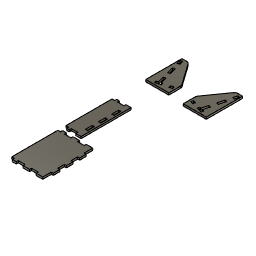
socle_carte_makers_quest_v5 (Autodesk Fusion 360 design; units mm, degrees)
Autodesk Fusion 360 part; units mm, degrees
sketch "Esquisse1" plane through (0, 0, 0) normal (0, 1, 0) x (1, 0, 0)
  line L0 (0, 0) -> (35, 0)
  line L1 (35, 0) -> (35, -55)
  line L2 (35, -55) -> (0, -55)
  line L3 (0, -55) -> (0, 0)
  line L4 (0, -55) -> (12.941, -6.7037)
  line L5 (0, -55) -> (50, -55) construction
  line L6 (12.941, -6.7037) -> (35, -12.6144)
  line L7 (12.941, -6.7037) -> (15.8387, -7.4802)
  line L8 (15.8387, -7.4802) -> (2.8978, -55.7765)
  line L9 (2.8978, -55.7765) -> (0, -55)
  line L10 (0, -55) -> (12.941, -6.7037)
  line L11 (35, -12.6144) -> (35.7765, -9.7166)
  line L12 (35.7765, -9.7166) -> (13.7176, -3.806)
  line L13 (13.7176, -3.806) -> (12.9412, -6.7038)
  line L14 (12.9412, -6.7038) -> (35, -12.6144)
  dimension "d1" = 35
  dimension "d2" = 55
  dimension "d3" = 75
  dimension "d4" = 50
  dimension "d5" = 3
  dimension "d6" = 50
  dimension "d7" = 22.8372
  dimension "d8" = 3
  dimension "d9" = 22.837
  constraint horizontal L0
  constraint vertical L1
  constraint horizontal L2
  constraint vertical L3
  constraint coincident L0.start L3.end
  constraint horizontal L5
  constraint coincident L1 L6.end
  constraint perpendicular L4 L6
  constraint parallel L4 L10
  constraint parallel L6 L14
  measures "d1" distance of L0.start L0.end
  measures "d2" distance of L0.start L2.end
  measures "d3" angle of L4 L5
  measures "d4" distance of L2.end L4.end
  measures "d5" distance of L4.end L7.end
  measures "d6" distance of L4.end L2.end
  measures "d7" distance of L4.end L6.end
  measures "d8" distance of L6.end L11.end
  measures "d9" distance of L6.end L13.end
extrude "Extrusion1" add sketch "Esquisse1" along normal blind 70 contours L1 L11 L12 | L1 L6 L7 L12 L13 L14 makes body 1
extrude "Extrusion2" add sketch "Esquisse1" along normal blind 70 separate body contours L2 L4 L6 L7 L8 L10 L14 | L2 L8 L9 makes body 2
extrude "Extrusion3" add sketch "Esquisse1" against normal blind 3 separate body contours L0 L1 L3 L4 L10 L12 L13 | L2 L4 L6 L7 L8 L10 L14 | L1 L6 L7 L12 L13 L14 | L1 L2 L6 L8 L14 makes body 3
copy_body "Copier/Coller des corps1" bodies 3 makes body 4
move_body "Déplacer1" bodies 4 to x (1, 0, 0) y (0, 1, 0) z (0, 0, 1) at (0, 73, 0)
extrude "Extrusion5" add 1 faces at (13.4587, 23.3333, 4.7719) along direction (-0.965926, 0, -0.258819) blind 3 on bodies 1 bodies 1
sketch "Esquisse2" plane through (-0.809, 0, 3.0194) normal (0.258819, 0, -0.965926) x (0, 1, 0)
  line L0 (0, 17.235) -> (0, 14.235)
  line L1 (0, 14.235) -> (70, 14.235)
  line L2 (70, 14.235) -> (70, 17.235)
  line L3 (70, 17.235) -> (0, 17.235)
  line L4 (0, 17.235) -> (10, 17.235) construction
  line L5 (10, 17.235) -> (10, 14.235) construction
  line L6 (10, 14.235) -> (0, 14.235) construction
  line L7 (0, 14.235) -> (0, 17.235) construction
  line L8 (70, 17.235) -> (60, 17.235) construction
  line L9 (60, 17.235) -> (60, 14.235) construction
  line L10 (60, 14.235) -> (70, 14.235) construction
  line L11 (70, 14.235) -> (70, 17.235) construction
  line L12 (10, 17.235) -> (20, 17.235)
  line L13 (20, 17.235) -> (20, 14.235)
  line L14 (20, 14.235) -> (10, 14.235)
  line L15 (10, 14.235) -> (10, 17.235)
  line L16 (60, 17.235) -> (50, 17.235)
  line L17 (50, 17.235) -> (50, 14.235)
  line L18 (50, 14.235) -> (60, 14.235)
  line L19 (60, 14.235) -> (60, 17.235)
  line L20 (20, 17.235) -> (30, 17.235) construction
  line L21 (30, 17.235) -> (30, 14.235) construction
  line L22 (30, 14.235) -> (20, 14.235) construction
  line L23 (20, 14.235) -> (20, 17.235) construction
  line L24 (30, 17.235) -> (40, 17.235)
  line L25 (40, 17.235) -> (40, 14.235)
  line L26 (40, 14.235) -> (30, 14.235)
  line L27 (30, 14.235) -> (30, 17.235)
  dimension "d20" = 10
  dimension "d21" = 10
  dimension "d22" = 10
  dimension "d23" = 10
  dimension "d24" = 10
  dimension "d25" = 10
  constraint horizontal L4
  constraint vertical L5
  constraint horizontal L6
  constraint vertical L7
  constraint coincident L0.start L3.end
  constraint horizontal L8
  constraint vertical L9
  constraint horizontal L10
  constraint vertical L11
  constraint coincident L2.end L3.start
  constraint horizontal L12
  constraint vertical L13
  constraint horizontal L14
  constraint vertical L15
  constraint horizontal L16
  constraint vertical L17
  constraint horizontal L18
  constraint vertical L19
  constraint horizontal L20
  constraint vertical L21
  constraint horizontal L22
  constraint vertical L23
  constraint horizontal L24
  constraint vertical L25
  constraint horizontal L26
  constraint vertical L27
  measures "d20" distance of L0.start L4.end
  measures "d21" distance of L2.end L8.end
  measures "d22" distance of L4.end L12.end
  measures "d23" distance of L8.end L16.end
  measures "d24" distance of L12.end L20.end
  measures "d25" distance of L20.end L24.end
extrude "Extrusion6" add sketch "Esquisse2" along normal blind 3 contours L1 L3 L12 L13 L14 L15 | L1 L3 L24 L25 L26 L27 | L1 L3 L16 L17 L18 L19 bodies 2
combine "Combiner1" operation cut target body 1 tool bodies 2 keep tools
sketch "Esquisse3" plane through (0, 70, 0) normal (0, 1, 0) x (-1, 0, 0)
  line L0 (-10.0434, 5.9273) -> (-35, 12.6144)
  line L1 (-35, 12.6144) -> (-35.7765, 9.7166)
  line L2 (-35.7765, 9.7166) -> (-10.8198, 3.0295)
  line L3 (-10.8198, 3.0295) -> (-10.0434, 5.9273)
  line L4 (-12.941, 6.7037) -> (0, 55)
  line L5 (0, 55) -> (-2.8978, 55.7765)
  line L6 (-2.8978, 55.7765) -> (-15.8387, 7.4802)
  line L7 (-15.8387, 7.4802) -> (-12.941, 6.7037)
  line L8 (-35, 12.6144) -> (-27.2726, 10.5439)
  line L9 (-27.2726, 10.5439) -> (-28.0491, 7.6461)
  line L10 (-28.0491, 7.6461) -> (-35.7765, 9.7166)
  line L11 (-35.7765, 9.7166) -> (-35, 12.6144)
  line L12 (-10.8198, 3.0295) -> (-18.5472, 5.1001)
  line L13 (0, 55) -> (-2.8978, 55.7765)
  line L14 (-2.5882, 45.3407) -> (0, 55)
  line L15 (-15.8387, 7.4802) -> (-12.941, 6.7037)
  line L16 (-12.941, 6.7037) -> (-10.3528, 16.363)
  line L17 (-10.3528, 16.363) -> (-13.2505, 17.1394)
  line L18 (-13.2505, 17.1394) -> (-15.8387, 7.4802)
  line L19 (-13.2505, 17.1394) -> (-10.3528, 16.363) construction
  line L20 (-2.8978, 55.7765) -> (-5.486, 46.1172)
  line L21 (-5.486, 46.1172) -> (-2.5882, 45.3407)
  line L22 (-8.0742, 36.4579) -> (-10.6623, 26.7987)
  line L23 (-10.6623, 26.7987) -> (-7.7646, 26.0222)
  line L24 (-8.0742, 36.4579) -> (-5.1764, 35.6815)
  line L25 (-5.1764, 35.6815) -> (-7.7646, 26.0222)
  line L26 (-10.8198, 3.0295) -> (-10.0434, 5.9273)
  line L27 (-10.0434, 5.9273) -> (-17.7708, 7.9979)
  line L28 (-17.7708, 7.9979) -> (-18.5472, 5.1001)
  line L29 (-3.9331, 51.9128) -> (-1.0353, 51.1363)
  line L30 (-31.1363, 11.5791) -> (-31.9128, 8.6814)
  point P0 (-8.0742, 36.4579)
  dimension "d28" = 8
  dimension "d29" = 3
  dimension "d30" = 8
  dimension "d32" = 3
  dimension "d33" = 10
  dimension "d34" = 3
  dimension "d35" = 10
  dimension "d38" = 3
  dimension "d42" = 10
  dimension "d43" = 10
  dimension "d44" = 10
  dimension "d45" = 8
  dimension "d50" = 3
  dimension "d51" = 4
  dimension "d52" = 4
  constraint coincident L0.end L1.start
  constraint parallel L2 L10
  constraint coincident L2.end L3.start
  constraint parallel L0 L12
  constraint coincident L4.end L5.start
  constraint coincident L6.end L7.start
  constraint parallel L4 L16
  constraint parallel L4 L14
  constraint perpendicular L13 L20
  constraint coincident L6 P0
  constraint coincident P0 L22.start
  constraint parallel L6 L22
  constraint coincident L4 L23.end
  constraint perpendicular L4 L23
  constraint coincident L4 L24.end
  constraint perpendicular L4 L24
  constraint coincident L0.start L3.end
  constraint perpendicular L26 L27
  constraint coincident L20 L29.start
  constraint coincident L6 L29.start
  constraint perpendicular L14 L29
  constraint perpendicular L20 L29
  constraint coincident L8 L30.start
  constraint coincident L0 L30.start
  constraint coincident L10 L30.end
  constraint perpendicular L8 L30
  constraint perpendicular L10 L30
  measures "d28" distance of L0.end L8.end
  measures "d29" distance of L0.end L1.end
  measures "d30" distance of L2.end L12.end
  measures "d32" distance of L4.end L5.end
  measures "d33" distance of L4.end L14.start
  measures "d34" distance of L6.end L4.start
  measures "d35" distance of L6.end L17.end
  measures "d38" distance of L17.end L16.end
  measures "d42" distance of L5.end L20.end
  measures "d43" distance of L20.end P0
  measures "d44" distance of P0 L22.end
  measures "d45" distance of L0.start L27.end
  measures "d50" distance of L29.start L29.end
  measures "d51" distance of L5.end L29.start
  measures "d52" distance of L0.end L30.start
extrude "Extrusion7" add sketch "Esquisse3" along normal blind 3 contours L0 L2 L3 L7 L12 L15 L26 L27 L28 | L0 L2 L8 L9 L10 L30 bodies 1
extrude "Extrusion8" add sketch "Esquisse3" along normal blind 3 contours L0 L4 L6 L7 L15 L16 L17 L18 L27 | L4 L6 L22 L23 L24 L25 | L4 L6 L14 L20 L21 L29 bodies 2
ref_plane "Plan de construction1" through (10.5076, 35, 21.5808) normal (0, 1, 0) x (0, 0, 1)
mirror "Symétrie miroir1" about plane through (10.5076, 35, 21.5808) normal (0, 1, 0) of "Extrusion7"
mirror "Symétrie miroir2" about plane through (10.5076, 35, 21.5808) normal (0, 1, 0) of "Extrusion8"
combine "Combiner2" operation cut target body 4 tool bodies 2 1 keep tools
combine "Combiner3" operation cut target body 3 tool bodies 2 1 keep tools
sketch "Esquisse4" plane through (0, 73, 0) normal (0, 1, 0) x (-1, 0, 0)
  line L0 (0, 55) -> (-35, 55)
  line L1 (-35, 55) -> (-35, 0)
  line L2 (-35, 0) -> (0, 0)
  line L3 (0, 0) -> (0, 55)
  line L4 (-12.941, 6.7037) -> (-10.0434, 5.9273)
  line L5 (-10.0434, 5.9273) -> (-10.8198, 3.0295)
  line L6 (-10.8198, 3.0295) -> (-18.5472, 5.1001)
  line L7 (-18.5472, 5.1001) -> (-17.7708, 7.9979)
  line L8 (-17.7708, 7.9979) -> (-15.8387, 7.4802)
  line L9 (-15.8387, 7.4802) -> (-13.2505, 17.1394)
  line L10 (-13.2505, 17.1394) -> (-10.3528, 16.363)
  line L11 (-10.3528, 16.363) -> (-12.941, 6.7037)
  line L12 (-7.7646, 26.0222) -> (-10.6623, 26.7987)
  line L13 (-10.6623, 26.7987) -> (-8.0742, 36.4579)
  line L14 (-8.0742, 36.4579) -> (-5.1764, 35.6815)
  line L15 (-5.1764, 35.6815) -> (-7.7646, 26.0222)
  line L16 (-2.5882, 45.3407) -> (-5.486, 46.1172)
  line L17 (-5.486, 46.1172) -> (-3.9331, 51.9128)
  line L18 (-3.9331, 51.9128) -> (-1.0353, 51.1363)
  line L19 (-1.0353, 51.1363) -> (-2.5882, 45.3407)
  line L20 (-31.9128, 8.6814) -> (-31.1363, 11.5791)
  line L21 (-31.1363, 11.5791) -> (-27.2726, 10.5439)
  line L22 (-27.2726, 10.5439) -> (-28.0491, 7.6461)
  line L23 (-28.0491, 7.6461) -> (-31.9128, 8.6814)
  line L24 (-10, 55) -> (-35, 19.6144)
  line L25 (-31.9128, 8.6814) -> (-31.1363, 11.5791)
  line L26 (-31.1363, 11.5791) -> (-35, 12.6144)
  line L27 (-35, 12.6144) -> (-35.7765, 9.7166)
  line L28 (-35.7765, 9.7166) -> (-31.9128, 8.6814)
  dimension "d58" = 10
  dimension "d59" = 7
  constraint coincident L0 L24.start
  constraint coincident L1 L24.end
  measures "d58" distance of L0.start L24.start
  measures "d59" distance of L24.end L26.end
extrude "Extrusion9" cut sketch "Esquisse4" against normal blind 80 contours L0 L1 L24 bodies 3 4
fillet "Congé1" radius 5 2 edges at (10, -1.5, 55) (10, 71.5, 55) on bodies 3 4
fillet "Congé1" radius 5 2 edges at (35, -1.5, 19.6144) (35, 71.5, 19.6144) on bodies 3 4
sketch "Esquisse5" plane through (0, 0, 0) normal (0, 0, 1) x (1, 0, 0)
  line L0 (-58.5004, 185.433) -> (-267.5004, 185.433)
  line L1 (-267.5004, 185.433) -> (-267.5004, -120.567)
  line L2 (-267.5004, -120.567) -> (-58.5004, -120.567)
  line L3 (-58.5004, -120.567) -> (-58.5004, 185.433)
  dimension "d66" = 209
  dimension "d67" = 306
  constraint horizontal L0
  constraint vertical L1
  constraint horizontal L2
  constraint vertical L3
  measures "d66" distance of L0.start L0.end
  measures "d67" distance of L0.start L2.end
copy_body "Corps->Comp1" bodies 1 removing the originals makes body 5 in component "Component'"
copy_body "Corps->Comp2" bodies 3 removing the originals makes body 6 in component "Component''"
copy_body "Corps->Comp3" bodies 4 removing the originals makes body 7 in component "Component'''"
copy_body "Corps->Comp4" bodies 2 removing the originals makes body 8 in component "Component''''"
other "Réorganiser1"
sketch "Esquisse1 (2)" plane through (-0.809, 0, 3.0194) normal (-0.258819, 0, 0.965926) x (0, -1, 0) in component "Component'"
  line L0 (-10, 14.235) -> (-20, 14.235)
  line L1 (-20, 14.235) -> (-20, 17.235)
  line L2 (-20, 17.235) -> (-10, 17.235)
  line L3 (-10, 17.235) -> (-10, 14.235)
  line L4 (-30, 14.235) -> (-40, 14.235)
  line L5 (-40, 14.235) -> (-40, 17.235)
  line L6 (-40, 17.235) -> (-30, 17.235)
  line L7 (-30, 17.235) -> (-30, 14.235)
  line L8 (-50, 14.235) -> (-60, 14.235)
  line L9 (-60, 14.235) -> (-60, 17.235)
  line L10 (-60, 17.235) -> (-50, 17.235)
  line L11 (-50, 17.235) -> (-50, 14.235)
  line L12 (0, 19.2353) -> (0, 29.0723)
  line L13 (0, 29.0723) -> (3, 29.0723)
  line L14 (3, 29.0723) -> (3, 33.0723)
  line L15 (3, 33.0723) -> (0, 33.0723)
  line L16 (0, 33.0723) -> (0, 37.0723)
  line L17 (0, 37.0723) -> (-70, 37.0723)
  line L18 (-70, 37.0723) -> (-70, 33.0723)
  line L19 (-70, 33.0723) -> (-73, 33.0723)
  line L20 (-73, 33.0723) -> (-73, 29.0723)
  line L21 (-73, 29.0723) -> (-70, 29.0723)
  line L22 (-70, 29.0723) -> (-70, 19.2353)
  line L23 (-70, 19.2353) -> (-73, 19.2353)
  line L24 (-73, 19.2353) -> (-73, 11.2353)
  line L25 (-73, 11.2353) -> (3, 11.2353)
  line L26 (3, 11.2353) -> (3, 19.2353)
  line L27 (3, 19.2353) -> (0, 19.2353)
sketch "Esquisse1 (3)" plane through (0, -3, 0) normal (0, -1, 0) x (1, 0, 0) in component "Component''"
  arc A0 (35, 18.0263) -> (34.0836, 20.9114) centre (30, 18.0263) ccw
  line L0 (34.0836, 20.9114) -> (11.4942, 52.8851)
  arc A1 (11.4942, 52.8851) -> (7.4105, 55) centre (7.4105, 50) ccw
  line L1 (7.4105, 55) -> (0, 55)
  line L2 (0, 55) -> (0, 0)
  line L3 (0, 0) -> (35, 0)
  line L4 (35, 0) -> (35, 18.0263)
  line L5 (10.6623, 26.7987) -> (7.7646, 26.0222)
  line L6 (7.7646, 26.0222) -> (5.1764, 35.6815)
  line L7 (5.1764, 35.6815) -> (8.0742, 36.4579)
  line L8 (8.0742, 36.4579) -> (10.6623, 26.7987)
  line L9 (5.486, 46.1172) -> (2.5882, 45.3407)
  line L10 (2.5882, 45.3407) -> (1.0353, 51.1363)
  line L11 (1.0353, 51.1363) -> (3.9331, 51.9128)
  line L12 (3.9331, 51.9128) -> (5.486, 46.1172)
  line L13 (31.1363, 11.5791) -> (31.9128, 8.6814)
  line L14 (31.9128, 8.6814) -> (28.0491, 7.6461)
  line L15 (28.0491, 7.6461) -> (27.2726, 10.5439)
  line L16 (27.2726, 10.5439) -> (31.1363, 11.5791)
  line L17 (10.0434, 5.9273) -> (12.941, 6.7037)
  line L18 (12.941, 6.7037) -> (10.3528, 16.363)
  line L19 (10.3528, 16.363) -> (13.2505, 17.1394)
  line L20 (13.2505, 17.1394) -> (15.8387, 7.4802)
  line L21 (15.8387, 7.4802) -> (17.7708, 7.9979)
  line L22 (17.7708, 7.9979) -> (18.5472, 5.1001)
  line L23 (18.5472, 5.1001) -> (10.8198, 3.0295)
  line L24 (10.8198, 3.0295) -> (10.0434, 5.9273)
sketch "Esquisse1 (4)" plane through (16.6478, 0, 4.4608) normal (0.965926, 0, 0.258819) x (0, 1, 0) in component "Component''''"
  line L0 (-3, 3.1259) -> (10, 3.1259)
  line L1 (10, 3.1259) -> (10, 0.1259)
  line L2 (10, 0.1259) -> (20, 0.1259)
  line L3 (20, 0.1259) -> (20, 3.1259)
  line L4 (20, 3.1259) -> (30, 3.1259)
  line L5 (30, 3.1259) -> (30, 0.1259)
  line L6 (30, 0.1259) -> (40, 0.1259)
  line L7 (40, 0.1259) -> (40, 3.1259)
  line L8 (40, 3.1259) -> (50, 3.1259)
  line L9 (50, 3.1259) -> (50, 0.1259)
  line L10 (50, 0.1259) -> (60, 0.1259)
  line L11 (60, 0.1259) -> (60, 3.1259)
  line L12 (60, 3.1259) -> (73, 3.1259)
  line L13 (73, 3.1259) -> (73, 13.1259)
  line L14 (73, 13.1259) -> (70, 13.1259)
  line L15 (70, 13.1259) -> (70, 23.1259)
  line L16 (70, 23.1259) -> (73, 23.1259)
  line L17 (73, 23.1259) -> (73, 33.1259)
  line L18 (73, 33.1259) -> (70, 33.1259)
  line L19 (70, 33.1259) -> (70, 43.1259)
  line L20 (70, 43.1259) -> (73, 43.1259)
  line L21 (73, 43.1259) -> (73, 49.1259)
  line L22 (73, 49.1259) -> (70, 49.1259)
  line L23 (70, 49.1259) -> (70, 53.1259)
  line L24 (70, 53.1259) -> (0, 53.1259)
  line L25 (0, 53.1259) -> (0, 49.1259)
  line L26 (0, 49.1259) -> (-3, 49.1259)
  line L27 (-3, 49.1259) -> (-3, 43.1259)
  line L28 (-3, 43.1259) -> (0, 43.1259)
  line L29 (0, 43.1259) -> (0, 33.1259)
  line L30 (0, 33.1259) -> (-3, 33.1259)
  line L31 (-3, 33.1259) -> (-3, 23.1259)
  line L32 (-3, 23.1259) -> (0, 23.1259)
  line L33 (0, 23.1259) -> (0, 13.1259)
  line L34 (0, 13.1259) -> (-3, 13.1259)
  line L35 (-3, 13.1259) -> (-3, 3.1259)
sketch "Esquisse1 (5)" plane through (0, 70, 0) normal (0, -1, 0) x (1, 0, 0) in component "Component'''"
  arc A0 (35, 18.0263) -> (34.0836, 20.9114) centre (30, 18.0263) ccw
  line L0 (34.0836, 20.9114) -> (11.4942, 52.8851)
  arc A1 (11.4942, 52.8851) -> (7.4105, 55) centre (7.4105, 50) ccw
  line L1 (7.4105, 55) -> (0, 55)
  line L2 (0, 55) -> (0, 0)
  line L3 (0, 0) -> (35, 0)
  line L4 (35, 0) -> (35, 18.0263)
  line L5 (1.0353, 51.1363) -> (3.9331, 51.9128)
  line L6 (3.9331, 51.9128) -> (5.486, 46.1172)
  line L7 (5.486, 46.1172) -> (2.5882, 45.3407)
  line L8 (2.5882, 45.3407) -> (1.0353, 51.1363)
  line L9 (5.1764, 35.6815) -> (8.0742, 36.4579)
  line L10 (8.0742, 36.4579) -> (10.6623, 26.7987)
  line L11 (10.6623, 26.7987) -> (7.7646, 26.0222)
  line L12 (7.7646, 26.0222) -> (5.1764, 35.6815)
  line L13 (28.0491, 7.6461) -> (27.2726, 10.5439)
  line L14 (27.2726, 10.5439) -> (31.1363, 11.5791)
  line L15 (31.1363, 11.5791) -> (31.9128, 8.6814)
  line L16 (31.9128, 8.6814) -> (28.0491, 7.6461)
  line L17 (18.5472, 5.1001) -> (10.8198, 3.0295)
  line L18 (10.8198, 3.0295) -> (10.0434, 5.9273)
  line L19 (10.0434, 5.9273) -> (12.941, 6.7037)
  line L20 (12.941, 6.7037) -> (10.3528, 16.363)
  line L21 (10.3528, 16.363) -> (13.2505, 17.1394)
  line L22 (13.2505, 17.1394) -> (15.8387, 7.4802)
  line L23 (15.8387, 7.4802) -> (17.7708, 7.9979)
  line L24 (17.7708, 7.9979) -> (18.5472, 5.1001)
move_body "Déplacer1'" bodies 7 to x (1, 0, 0) y (0, -1, 0) z (0, 0, -1) at (-45.3829, 140, 0) in component "Component'''"
sketch "Esquisse2 (2)" plane through (0, 67, 0) normal (0, -1, 0) x (1, 0, 0) in component "Component'''"
  arc A0 (-11.2993, -20.9114) -> (-10.3829, -18.0263) centre (-15.3829, -18.0263) ccw
  line L0 (-10.3829, -18.0263) -> (-10.3829, 0)
  line L1 (-10.3829, 0) -> (-45.3829, 0)
  line L2 (-45.3829, 0) -> (-45.3829, -55)
  line L3 (-45.3829, -55) -> (-37.9724, -55)
  arc A1 (-37.9724, -55) -> (-33.8887, -52.8851) centre (-37.9724, -50) ccw
  line L4 (-33.8887, -52.8851) -> (-11.2993, -20.9114)
  line L5 (-32.442, -6.7037) -> (-35.3395, -5.9273)
  line L6 (-35.3395, -5.9273) -> (-34.5631, -3.0295)
  line L7 (-34.5631, -3.0295) -> (-26.8357, -5.1001)
  line L8 (-26.8357, -5.1001) -> (-27.6121, -7.9979)
  line L9 (-27.6121, -7.9979) -> (-29.5442, -7.4802)
  line L10 (-29.5442, -7.4802) -> (-32.1324, -17.1394)
  line L11 (-32.1324, -17.1394) -> (-35.0301, -16.363)
  line L12 (-35.0301, -16.363) -> (-32.442, -6.7037)
  line L13 (-37.6183, -26.0222) -> (-34.7206, -26.7987)
  line L14 (-34.7206, -26.7987) -> (-37.3087, -36.4579)
  line L15 (-37.3087, -36.4579) -> (-40.2065, -35.6815)
  line L16 (-40.2065, -35.6815) -> (-37.6183, -26.0222)
  line L17 (-42.7947, -45.3407) -> (-39.8969, -46.1172)
  line L18 (-39.8969, -46.1172) -> (-41.4499, -51.9128)
  line L19 (-41.4499, -51.9128) -> (-44.3476, -51.1363)
  line L20 (-44.3476, -51.1363) -> (-42.7947, -45.3407)
  line L21 (-13.4702, -8.6814) -> (-14.2466, -11.5791)
  line L22 (-14.2466, -11.5791) -> (-18.1103, -10.5439)
  line L23 (-18.1103, -10.5439) -> (-17.3339, -7.6461)
  line L24 (-17.3339, -7.6461) -> (-13.4702, -8.6814)
move_face "DécalerLesFaces1" offset -0.15 13 faces at (16.3564, 56.6667, 5.5483) (13.1998, 53.3333, 5.7378) (14.1657, 60, 5.9966) (15.1316, 50, 6.2554) (14.1657, 30, 5.9966) (14.1657, 10, 5.9966) (15.1316, 40, 6.2554) (15.1316, 20, 6.2554) (29.3894, 33.3333, 8.0052) (13.1998, 16.6667, 5.7378) (13.1998, 36.6667, 5.7378) (16.3564, 33.3333, 5.5483) (16.3564, 13.3333, 5.5483) on bodies 5 in component "Component'"
move_face "DécalerLesFaces1'" offset -0.15 20 faces at (10.561, -1, 3.9955) (11.2155, -2, 13.1432) (6.0391, -2, 32.4617) (2.0706, -1, 47.2726) (27.5314, -1, 9.5779) (15.9714, -2, 4.4099) (30.6249, -2, 8.3363) (9.6964, -1, 26.5399) (4.52, -1, 45.8584) (11.9751, -1, 6.4449) (17.1268, -1, 7.8253) (11.3187, -1, 16.6218) (7.1082, -1, 36.1991) (2.9671, -1, 51.6539) (28.5605, -1, 10.889) (4.4507, -1, 49.9809) (8.9369, -1, 33.2382) (14.976, -1, 10.6999) (18.2884, -2, 6.066) (31.3951, -1, 10.6132) on bodies 6 in component "Component''"
move_face "DécalerLesFaces1''" offset -0.15 20 faces at (-16.8224, 68, -10.889) (-13.9878, 69, -10.6132) (-27.0945, 68, -6.066) (-28.9002, 69, -7.6527) (-30.4069, 69, -10.6999) (-34.0642, 69, -16.6218) (-42.4158, 69, -51.6539) (-40.4146, 68, -48.0491) (-38.2747, 68, -36.1991) (-35.5833, 68, -30.0184) (-34.3737, 69, -6.1861) (-43.83, 69, -49.2044) (-38.4811, 68, -29.242) (-33.3047, 69, -9.9235) (-34.8219, 69, -3.9955) (-17.8515, 69, -9.5779) (-14.7581, 68, -8.3363) (-29.4115, 69, -4.4099) (-35.6865, 69, -26.5399) (-40.8629, 69, -45.8584) on bodies 7 in component "Component'''"
sketch "Esquisse2 (3)" plane through (-0.809, 0, 3.0194) normal (-0.258819, 0, 0.965926) x (0, -1, 0) in component "Component'"
  line L0 (-9.85, 14.085) -> (-20.15, 14.085)
  line L1 (-20.15, 14.085) -> (-20.15, 17.385)
  line L2 (-20.15, 17.385) -> (-9.85, 17.385)
  line L3 (-9.85, 17.385) -> (-9.85, 14.085)
  line L4 (-29.85, 14.085) -> (-40.15, 14.085)
  line L5 (-40.15, 14.085) -> (-40.15, 17.385)
  line L6 (-40.15, 17.385) -> (-29.85, 17.385)
  line L7 (-29.85, 17.385) -> (-29.85, 14.085)
  line L8 (-49.85, 14.085) -> (-60.15, 14.085)
  line L9 (-60.15, 14.085) -> (-60.15, 17.385)
  line L10 (-60.15, 17.385) -> (-49.85, 17.385)
  line L11 (-49.85, 17.385) -> (-49.85, 14.085)
  line L12 (0, 19.2353) -> (0, 29.0723)
  line L13 (0, 29.0723) -> (3, 29.0723)
  line L14 (3, 29.0723) -> (3, 33.0723)
  line L15 (3, 33.0723) -> (0, 33.0723)
  line L16 (0, 33.0723) -> (0, 37.0723)
  line L17 (0, 37.0723) -> (-70, 37.0723)
  line L18 (-70, 37.0723) -> (-70, 33.0723)
  line L19 (-70, 33.0723) -> (-73, 33.0723)
  line L20 (-73, 33.0723) -> (-73, 29.0723)
  line L21 (-73, 29.0723) -> (-70, 29.0723)
  line L22 (-70, 29.0723) -> (-70, 19.2353)
  line L23 (-70, 19.2353) -> (-73, 19.2353)
  line L24 (-73, 19.2353) -> (-73, 11.2353)
  line L25 (-73, 11.2353) -> (3, 11.2353)
  line L26 (3, 11.2353) -> (3, 19.2353)
  line L27 (3, 19.2353) -> (0, 19.2353)
sketch "Esquisse2 (4)" plane through (0, -3, 0) normal (0, -1, 0) x (1, 0, 0) in component "Component''"
  arc A0 (35, 18.0263) -> (34.0836, 20.9114) centre (30, 18.0263) ccw
  line L0 (34.0836, 20.9114) -> (11.4942, 52.8851)
  arc A1 (11.4942, 52.8851) -> (7.4105, 55) centre (7.4105, 50) ccw
  line L1 (7.4105, 55) -> (0, 55)
  line L2 (0, 55) -> (0, 0)
  line L3 (0, 0) -> (35, 0)
  line L4 (35, 0) -> (35, 18.0263)
  line L5 (10.8461, 26.6926) -> (7.6585, 25.8385)
  line L6 (7.6585, 25.8385) -> (4.9927, 35.7875)
  line L7 (4.9927, 35.7875) -> (8.1802, 36.6417)
  line L8 (8.1802, 36.6417) -> (10.8461, 26.6926)
  line L9 (5.6697, 46.0111) -> (2.4821, 45.157)
  line L10 (2.4821, 45.157) -> (0.8516, 51.2424)
  line L11 (0.8516, 51.2424) -> (4.0391, 52.0965)
  line L12 (4.0391, 52.0965) -> (5.6697, 46.0111)
  line L13 (31.2424, 11.7628) -> (32.0965, 8.5753)
  line L14 (32.0965, 8.5753) -> (27.943, 7.4624)
  line L15 (27.943, 7.4624) -> (27.0889, 10.6499)
  line L16 (27.0889, 10.6499) -> (31.2424, 11.7628)
  line L17 (9.8597, 6.0334) -> (12.7572, 6.8098)
  line L18 (12.7572, 6.8098) -> (10.1691, 16.469)
  line L19 (10.1691, 16.469) -> (13.3566, 17.3231)
  line L20 (13.3566, 17.3231) -> (15.9448, 7.6639)
  line L21 (15.9448, 7.6639) -> (17.8768, 8.1816)
  line L22 (17.8768, 8.1816) -> (18.7309, 4.994)
  line L23 (18.7309, 4.994) -> (10.7138, 2.8458)
  line L24 (10.7138, 2.8458) -> (9.8597, 6.0334)
component "Component'" placed x (-0.965926, 0, -0.258819) y (0, -1, 0) z (-0.258819, 0, 0.965926) at (-224.0782, 41.133, -0.1259)
component "Component''" placed x (1, 0, 0) y (0, 0, -1) z (0, 1, 0) at (-261.1504, 92.1949, 0)
component "Component'''" placed x (-1, 0, 0) y (0, 0, -1) z (0, -1, 0) at (-208.1504, 85.8449, 73)
component "Component''''" placed x (0.258819, 0, 0.965926) y (0, 1, 0) z (-0.965926, 0, 0.258819) at (-208.0245, -111.217, -14.235)
